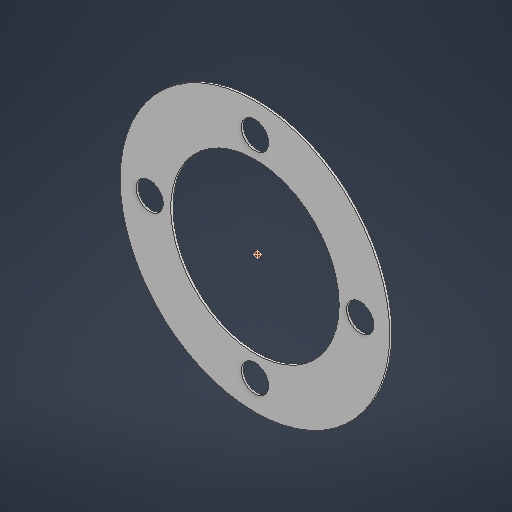
# Autodesk Inventor part: CylinderPacking
Saved by Autodesk Inventor 2025.4 (Build 294407000, 407)
## iProperties
Created: 2026-05-29
Part Number: CylinderPacking
Material: Generic
Document SubType Name: Modeling
Designer: VuQuan
Density: 1 g/cm^3
Appearance: Default
Author: VuQuan
Autodesk Inventor part; units mm, degrees
ref_plane "YZ Plane" through (0, 0, 0) normal (1, 0, 0) x (0, 1, 0)
ref_plane "XZ Plane" through (0, 0, 0) normal (0, 1, 0) x (-1, 0, 0)
ref_plane "XY Plane" through (0, 0, 0) normal (0, 0, 1) x (1, 0, 0)
sketch "Sketch1" plane through (0, 0, 0) normal (0, 0, 1) x (1, 0, 0)
  circle A0 centre (0, 0) radius 20
  circle A1 centre (0, 0) radius 25 construction
  circle A2 centre (0, 0) radius 32
  circle A3 centre (0, 25) radius 3.25
  circle A4 centre (-25, 0) radius 3.25
  circle A5 centre (0, -25) radius 3.25
  circle A6 centre (25, 0) radius 3.25
  dimension "d1" = 50
  dimension "d0" = 40
  dimension "d2" = 64
  dimension "d3" = 6.5
  dimension "d6" = 360
  constraints: 6 centre point, 3 coincident, 2 vertical alignment, 11 other
  measures "d0" diameter of A0
  measures "d2" diameter of A2
  measures "d3" diameter of A3
extrude "Extrusion1" add sketch "Sketch1" along normal blind 0.5
body "Solid1"
